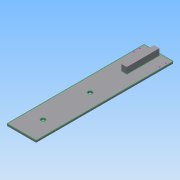
# Autodesk Inventor part: DaughterBoardOutline
Saved by Autodesk Inventor 2013 (Build 170138000, 138)
## iProperties
Created: 2012-08-25
Part Number: DaughterBoardOutline
Material: Generic
Document SubType Name: Modeling
Designer: henry
Density: 1 g/cm^3
Author: henry
Autodesk Inventor part; units mm, degrees
ref_plane "YZ Plane" through (0, 0, 0) normal (1, 0, 0) x (0, 1, 0)
ref_plane "XZ Plane" through (0, 0, 0) normal (0, 1, 0) x (-1, 0, 0)
ref_plane "XY Plane" through (0, 0, 0) normal (0, 0, 1) x (1, 0, 0)
sketch "Sketch1" plane through (0, 0, 0) normal (0, 1, 0) x (-1, 0, 0)
  line L0 (-10.795, -50.8) -> (10.795, -50.8)
  line L1 (10.795, -50.8) -> (10.795, 50.8)
  line L2 (10.795, 50.8) -> (-10.795, 50.8)
  line L3 (-10.795, 50.8) -> (-10.795, -50.8)
  line L4 (-10.795, -50.8) -> (10.795, 50.8) construction
  line L5 (10.795, -50.8) -> (-10.795, 50.8) construction
  point P0 (0, 0)
  dimension "d0" = 21.59
  dimension "d2" = 101.6
  constraints: 12 end point, 2 midpoint, 2 parallel, 1 horizontal, 1 perpendicular
  measures "d0" distance of L1.end L2.end
  measures "d2" distance of L2.end L0.start
extrude "Extrusion1" add sketch "Sketch1" along normal blind 1.5875
sketch "Sketch2" plane through (0, 1.5875, 0) normal (0, 1, 0) x (1, 0, 0)
  line L0 (10.795, 50.8) -> (-10.795, 50.8) projected
  line L1 (-10.795, -50.8) -> (10.795, -50.8) projected
  line L2 (0, 50.8) -> (0, -42.8954)
  line L3 (-2, 25.33) -> (2, 25.33)
  line L4 (2, 25.33) -> (2, 49.53)
  line L5 (2, 49.53) -> (-2, 49.53)
  line L6 (-2, 49.53) -> (-2, 25.33)
  line L7 (-2, 25.33) -> (2, 49.53) construction
  line L8 (2, 25.33) -> (-2, 49.53) construction
  point P0 (0, 0)
  point P1 (0, 37.43)
  dimension "d5" = 4
  dimension "d8" = 24.2
  dimension "d20" = 1.27
  constraints: 14 end point, 3 midpoint, 2 parallel, 2 perpendicular, 1 horizontal, 1 point on line
  measures "d5" distance of L4.end L5.end
  measures "d8" distance between parallel lines of L3 L5
  measures "d20" distance between parallel lines of L0 L5
extrude "Extrusion2" add sketch "Sketch2" along normal blind 4.55
sketch "Sketch3" plane through (0, 1.5875, 0) normal (0, 1, 0) x (1, 0, 0)
  line L0 (10.795, 50.8) -> (-10.795, 50.8) projected
  point P0 (0, -34.925)
  point P1 (0, 0)
  point P2 (0, 15.875)
  dimension "d21" = 34.925
  dimension "d22" = 50.8
  measures "d21" distance from line of L0 point (0, 15.875)
  measures "d22" distance of point (0, 15.875) point (0, -34.925)
hole "Hole1" at (0, 1.5875, 34.925) at (0, 1.5875, 0) direction (0, -1, 0) diameter 3.175 end through all
sketch "Sketch4" plane through (0, 1.5875, 0) normal (0, 1, 0) x (1, 0, 0)
  circle A0 centre (0, -34.925) radius 1.5875 projected
  circle A1 centre (0, 0) radius 1.5875 projected
  line L0 (-2, 25.33) -> (-2, 49.53) projected
  line L1 (-2, 49.53) -> (2, 49.53) projected
  line L2 (2, 49.53) -> (2, 25.33) projected
  line L3 (2, 25.33) -> (-2, 25.33) projected
  line L4 (10.795, 50.8) -> (-10.795, 50.8) projected
  line L5 (-10.795, 50.8) -> (-10.795, -50.8) projected
  line L6 (-10.795, -50.8) -> (10.795, -50.8) projected
  line L7 (10.795, -50.8) -> (10.795, 50.8) projected
  point P0 (-9.525, 46.675)
  point P1 (9.525, 46.675)
  point P2 (9.525, 42.225)
  point P3 (-9.525, 42.225)
  constraints: 2 other
body "Solid1"
